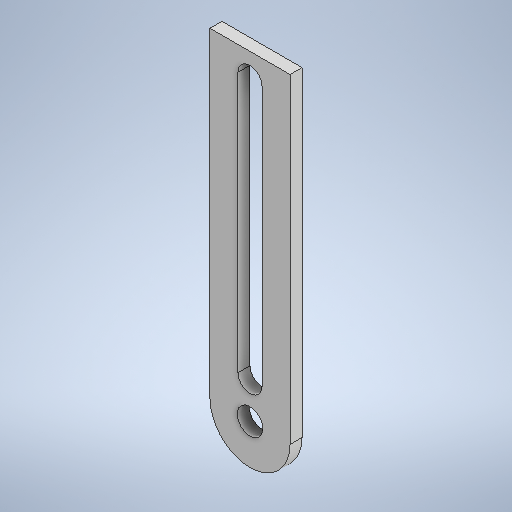
# Autodesk Inventor part: kosinopich
Saved by Autodesk Inventor 2025.1 (Build 291241000, 241)
## iProperties
Created: 2024-09-01
Part Number: kosinopich
Material: 一般
Document SubType Name: Modeling
Designer: right
Density: 1 g/cm^3
Appearance: 既定
Author: right
Autodesk Inventor part; units mm, degrees
ref_plane "YZ Plane" through (0, 0, 0) normal (1, 0, 0) x (0, 1, 0)
ref_plane "XZ Plane" through (0, 0, 0) normal (0, 1, 0) x (-1, 0, 0)
ref_plane "XY Plane" through (0, 0, 0) normal (0, 0, 1) x (1, 0, 0)
sketch "スケッチ1" plane through (0, 0, 0) normal (0, 0, 1) x (1, 0, 0)
  circle A0 centre (0, 0) radius 1.6
  circle A1 centre (0, 0) radius 5
  line L0 (-5, 0) -> (-5, 40)
  line L1 (-5, 40) -> (5, 40)
  line L2 (5, 40) -> (5, 0)
  dimension "d0" = 3.2
  dimension "d1" = 10
  dimension "d2" = 40
  constraints: 6 end point, 2 centre point, 2 coincident, 2 point on circle, 2 tangent, 2 vertical, 1 perpendicular
  measures "d0" diameter of A0
  measures "d1" diameter of A1
  measures "d2" distance from line of point (0, 0) L1
extrude "押し出し1" add sketch "スケッチ1" along normal blind 1.5
sketch "スケッチ2" plane through (0, 0, 1.5) normal (0, 0, 1) x (1, 0, 0)
  circle A0 centre (0, 0) radius 1.6 projected
  circle A1 centre (0, 0) radius 3
  circle A2 centre (0, 4.5) radius 1.5
  circle A3 centre (0, 37) radius 1.5
  line L0 (5, 40) -> (-5, 40) projected
  line L1 (1.5, 37) -> (1.5, 4.5)
  line L2 (-1.5, 37) -> (-1.5, 4.5)
  dimension "d5" = 6
  dimension "d6" = 3
  dimension "d7" = 3
  constraints: 5 tangent, 4 end point, 4 point on circle, 3 centre point, 2 vertical alignment, 1 coincident, 1 equal radius
  measures "d5" diameter of A1
  measures "d6" diameter of A2
  measures "d7" distance from line of L0 A3.centre
extrude "押し出し2" cut sketch "スケッチ2" against normal through all contours A2 | L2 A3 L1 A2 | A3
